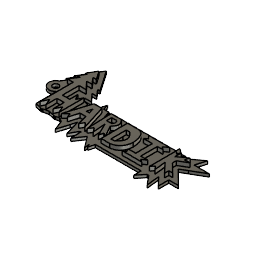
hackclub_day3 (Autodesk Fusion 360 design; units mm, degrees)
part number: 2025-12-19-10-28-26-184
Autodesk Fusion 360 part; units mm, degrees
sketch "Sketch2" plane through (0, 0, 0) normal (0, 0, 1) x (1, 0, 0)
  line L0 (23.8066, -11.3705) -> (28.9661, -18.9111)
  line L1 (28.9661, -18.9111) -> (32.7901, -24.5)
  line L2 (32.7901, -24.5) -> (30.8533, -24.5)
  line L3 (30.8533, -24.5) -> (35.4835, -29.9238)
  line L4 (35.4835, -29.9238) -> (31.3674, -29.9238)
  line L5 (31.3674, -29.9238) -> (31.9281, -30.5202)
  line L6 (31.9281, -30.5202) -> (37.5851, -36.5384)
  line L7 (37.5851, -36.5384) -> (31.3984, -36.5384)
  line L8 (31.3984, -36.5384) -> (32.4268, -38.3381)
  line L9 (32.4268, -38.3381) -> (32.6557, -38.739)
  line L10 (32.6557, -38.739) -> (38.0566, -40.1103)
  line L11 (38.0566, -40.1103) -> (38.0566, -44.6386)
  line L12 (38.0566, -44.6386) -> (39.8071, -39.0438)
  line L13 (39.8071, -39.0438) -> (40.5908, -36.5384)
  line L14 (40.5908, -36.5384) -> (45.497, -36.5384)
  line L15 (45.497, -36.5384) -> (46.8807, -31.8775)
  line L16 (46.8807, -31.8775) -> (48.1917, -36.5384)
  line L17 (48.1917, -36.5384) -> (52.7203, -36.5384)
  line L18 (52.7203, -36.5384) -> (53.504, -39.0438)
  line L19 (53.504, -39.0438) -> (54.5409, -42.3579)
  line L20 (54.5409, -42.3579) -> (54.4632, -40.2418)
  line L21 (54.4632, -40.2418) -> (54.3269, -36.5384)
  line L22 (54.3269, -36.5384) -> (68.5789, -36.5384)
  line L23 (68.5789, -36.5384) -> (68.7483, -36.7197)
  line L24 (68.7483, -36.7197) -> (68.7483, -36.5384)
  line L25 (68.7483, -36.5384) -> (79.7116, -36.5384)
  spline S0 degree 3 poles (79.7116, -36.5384) (80.9546, -36.4376) (82.1108, -36.5411) (83.1757, -36.8107) knots 0 0 0 0 1 1 1 1
  line L26 (83.1757, -36.8107) -> (82.9429, -36.5384)
  line L27 (82.9429, -36.5384) -> (110.6847, -36.5384)
  line L28 (110.6847, -36.5384) -> (110.6847, -33.1248)
  line L29 (110.6847, -33.1248) -> (115.4115, -36.5384)
  line L30 (115.4115, -36.5384) -> (119.5483, -36.5384)
  line L31 (119.5483, -36.5384) -> (117.5189, -38.0603)
  line L32 (117.5189, -38.0603) -> (117.8817, -38.3222)
  line L33 (117.8817, -38.3222) -> (120.0325, -38.83)
  line L34 (120.0325, -38.83) -> (123.5387, -36.2913)
  line L35 (123.5387, -36.2913) -> (131.9062, -30.2321)
  line L36 (131.9062, -30.2321) -> (129.3109, -39.3166)
  line L37 (129.3109, -39.3166) -> (142.5043, -39.3166)
  line L38 (142.5043, -39.3166) -> (130.9952, -45.9798)
  line L39 (130.9952, -45.9798) -> (125.3969, -49.2207)
  line L40 (125.3969, -49.2207) -> (131.7088, -55.4217)
  line L41 (131.7088, -55.4217) -> (137.9379, -61.5416)
  line L42 (137.9379, -61.5416) -> (129.4701, -61.5416)
  line L43 (129.4701, -61.5416) -> (129.4701, -70.7065)
  line L44 (129.4701, -70.7065) -> (123.2927, -64.117)
  line L45 (123.2927, -64.117) -> (122.6426, -63.4238)
  line L46 (122.6426, -63.4238) -> (123.8417, -74.6641)
  line L47 (123.8417, -74.6641) -> (117.3266, -66.7009)
  line L48 (117.3266, -66.7009) -> (115.9494, -66.7009)
  line L49 (115.9494, -66.7009) -> (110.6847, -73.1356)
  line L50 (110.6847, -73.1356) -> (110.6847, -66.7009)
  line L51 (110.6847, -66.7009) -> (71.0409, -66.7009)
  line L52 (71.0409, -66.7009) -> (69.7045, -72.0471)
  line L53 (69.7045, -72.0471) -> (68.3324, -69.2359)
  line L54 (68.3324, -69.2359) -> (68.7086, -73.7476)
  line L55 (68.7086, -73.7476) -> (61.4852, -64.1165)
  line L56 (61.4852, -64.1165) -> (55.6583, -72.7043)
  line L57 (55.6583, -72.7043) -> (55.3135, -63.3428)
  line L58 (55.3135, -63.3428) -> (54.4314, -63.8315)
  line L59 (54.4314, -63.8315) -> (50.4209, -70.8501)
  line L60 (50.4209, -70.8501) -> (48.1118, -62.6412)
  line L61 (48.1118, -62.6412) -> (46.695, -57.6032)
  line L62 (46.695, -57.6032) -> (45.185, -62.6904)
  line L63 (45.185, -62.6904) -> (42.2312, -72.64)
  line L64 (42.2312, -72.64) -> (38.9268, -64.2289)
  line L65 (38.9268, -64.2289) -> (35.6341, -62.1964)
  line L66 (35.6341, -62.1964) -> (32.7348, -62.8216)
  line L67 (32.7348, -62.8216) -> (32.5504, -63.2095)
  line L68 (32.5504, -63.2095) -> (31.7622, -63.0314)
  line L69 (31.7622, -63.0314) -> (31.2304, -63.1463)
  line L70 (31.2304, -63.1463) -> (31.1118, -62.8843)
  line L71 (31.1118, -62.8843) -> (26.1822, -61.7704)
  line L72 (26.1822, -61.7704) -> (21.5773, -62.6674)
  line L73 (21.5773, -62.6674) -> (21.2755, -63.2711)
  line L74 (21.2755, -63.2711) -> (20.0102, -62.9724)
  line L75 (20.0102, -62.9724) -> (19.7968, -63.0142)
  line L76 (19.7968, -63.0142) -> (19.7555, -62.9124)
  line L77 (19.7555, -62.9124) -> (14.5087, -61.6738)
  line L78 (14.5087, -61.6738) -> (14.5087, -36.5384)
  line L79 (14.5087, -36.5384) -> (6.5268, -36.5384)
  line L80 (6.5268, -36.5384) -> (10.0449, -31.0412)
  line L81 (10.0449, -31.0412) -> (10.7599, -29.9238)
  line L82 (10.7599, -29.9238) -> (8.676, -29.9238)
  line L83 (8.676, -29.9238) -> (11.8231, -24.5475)
  line L84 (11.8231, -24.5475) -> (11.851, -24.5)
  line L85 (11.851, -24.5) -> (10.2979, -24.5)
  line L86 (10.2979, -24.5) -> (13.4018, -19.1385)
  line L87 (13.4018, -19.1385) -> (17.7675, -11.5979)
  line L88 (17.7675, -11.5979) -> (20.6068, -6.6938)
  line L89 (20.6068, -6.6938) -> (23.8066, -11.3705)
  spline S1 degree 3 poles (80.5222, -52.3415) (80.5257, -52.3163) (80.5257, -52.3055) (80.5259, -52.3089) knots 0 0 0 0 1 1 1 1
  spline S2 degree 3 poles (80.5259, -52.3089) (80.5257, -52.3076) (80.5246, -52.3012) (80.5222, -52.2893) knots 0 0 0 0 1 1 1 1
  line L90 (80.5222, -52.2893) -> (80.5222, -52.3415)
  circle A0 centre (19.8343, -1.9154) radius 8.0516
  circle A1 centre (19.8343, -1.9154) radius 4.4627
  constraint concentric A0 A1
extrude "Extrude1" add sketch "Sketch2" along normal blind 2.5 contours L0 L1 L2 L3 L4 L5 L6 L7 L8 L9 L10 L11 L12 L13 L14 L15 L16 L17 L18 L19 L20 L21 L22 L23 L24 L25 S0 L26 L27 L28 L29 L30 L31 L32 L33 L34 L35 L36 L37 L38 L39 L40 L41 L42 L43 L44 L45 L46 L47 L48 L49 L50 L51 L52 L53 L54 L55 L56 L57 L58 L59 L60 L61 L62 L63 L64 L65 L66 L67 L68 L69 L70 L71 L72 L73 L74 L75 L76 L77 L78 L79 L80 L81 L82 L83 L84 L85 L86 L87 L88 L89 A0 | L88 L89 A0 picked at (20.9602, -8.7956)
sketch "Sketch3" plane through (0, 0, 2.5) normal (0, 0, 1) x (-1, 0, 0)
  line L0 (-80.5222, 52.3415) -> (-80.5222, 52.2893)
  spline S0 degree 3 poles (-80.5222, 52.2893) (-80.5244, 52.3) (-80.5254, 52.3062) (-80.5258, 52.3083) knots -1 -1 -1 -1 -0.105948 -0.105948 -0.105948 -0.105948
  spline S1 degree 3 poles (-80.5258, 52.3083) (-80.5256, 52.309) (-80.5252, 52.32) (-80.5222, 52.3415) knots -0.853043 -0.853043 -0.853043 -0.853043 0 0 0 0
  line L1 (-20.6068, 6.6938) -> (-17.7675, 11.5979)
  line L2 (-17.7675, 11.5979) -> (-13.4018, 19.1385)
  line L3 (-13.4018, 19.1385) -> (-10.2979, 24.5)
  line L4 (-10.2979, 24.5) -> (-11.851, 24.5)
  line L5 (-11.851, 24.5) -> (-11.8231, 24.5475)
  line L6 (-11.8231, 24.5475) -> (-8.676, 29.9238)
  line L7 (-8.676, 29.9238) -> (-10.7599, 29.9238)
  line L8 (-10.7599, 29.9238) -> (-10.0449, 31.0412)
  line L9 (-10.0449, 31.0412) -> (-6.5268, 36.5384)
  line L10 (-6.5268, 36.5384) -> (-14.5087, 36.5384)
  line L11 (-14.5087, 36.5384) -> (-14.5087, 61.6738)
  line L12 (-14.5087, 61.6738) -> (-19.7555, 62.9124)
  line L13 (-19.7555, 62.9124) -> (-19.7968, 63.0142)
  line L14 (-19.7968, 63.0142) -> (-20.0102, 62.9724)
  line L15 (-20.0102, 62.9724) -> (-21.2755, 63.2711)
  line L16 (-21.2755, 63.2711) -> (-21.5773, 62.6674)
  line L17 (-21.5773, 62.6674) -> (-26.1822, 61.7704)
  line L18 (-26.1822, 61.7704) -> (-31.1118, 62.8843)
  line L19 (-31.1118, 62.8843) -> (-31.2304, 63.1463)
  line L20 (-31.2304, 63.1463) -> (-31.7622, 63.0314)
  line L21 (-31.7622, 63.0314) -> (-32.5504, 63.2095)
  line L22 (-32.5504, 63.2095) -> (-32.7348, 62.8216)
  line L23 (-32.7348, 62.8216) -> (-35.6341, 62.1964)
  line L24 (-35.6341, 62.1964) -> (-38.9268, 64.2289)
  line L25 (-38.9268, 64.2289) -> (-42.2312, 72.64)
  line L26 (-42.2312, 72.64) -> (-45.185, 62.6904)
  line L27 (-45.185, 62.6904) -> (-46.695, 57.6032)
  line L28 (-46.695, 57.6032) -> (-48.1118, 62.6412)
  line L29 (-48.1118, 62.6412) -> (-50.4209, 70.8501)
  line L30 (-50.4209, 70.8501) -> (-54.4314, 63.8315)
  line L31 (-54.4314, 63.8315) -> (-55.3135, 63.3428)
  line L32 (-55.3135, 63.3428) -> (-55.6583, 72.7043)
  line L33 (-55.6583, 72.7043) -> (-61.4852, 64.1165)
  line L34 (-61.4852, 64.1165) -> (-68.7086, 73.7476)
  line L35 (-68.7086, 73.7476) -> (-68.3324, 69.2359)
  line L36 (-68.3324, 69.2359) -> (-69.7045, 72.0471)
  line L37 (-69.7045, 72.0471) -> (-71.0409, 66.7009)
  line L38 (-71.0409, 66.7009) -> (-110.6847, 66.7009)
  line L39 (-110.6847, 66.7009) -> (-110.6847, 73.1356)
  line L40 (-110.6847, 73.1356) -> (-115.9494, 66.7009)
  line L41 (-115.9494, 66.7009) -> (-117.3266, 66.7009)
  line L42 (-117.3266, 66.7009) -> (-123.8417, 74.6641)
  line L43 (-123.8417, 74.6641) -> (-122.6426, 63.4238)
  line L44 (-122.6426, 63.4238) -> (-123.2927, 64.117)
  line L45 (-123.2927, 64.117) -> (-129.4701, 70.7065)
  line L46 (-129.4701, 70.7065) -> (-129.4701, 61.5416)
  line L47 (-129.4701, 61.5416) -> (-137.9379, 61.5416)
  line L48 (-137.9379, 61.5416) -> (-131.7088, 55.4217)
  line L49 (-131.7088, 55.4217) -> (-125.3969, 49.2207)
  line L50 (-125.3969, 49.2207) -> (-130.9952, 45.9798)
  line L51 (-130.9952, 45.9798) -> (-142.5043, 39.3166)
  line L52 (-142.5043, 39.3166) -> (-129.3109, 39.3166)
  line L53 (-129.3109, 39.3166) -> (-131.9062, 30.2321)
  line L54 (-131.9062, 30.2321) -> (-123.5387, 36.2913)
  line L55 (-123.5387, 36.2913) -> (-120.0325, 38.83)
  line L56 (-120.0325, 38.83) -> (-117.8817, 38.3222)
  line L57 (-117.8817, 38.3222) -> (-117.5189, 38.0603)
  line L58 (-117.5189, 38.0603) -> (-119.5483, 36.5384)
  line L59 (-119.5483, 36.5384) -> (-115.4115, 36.5384)
  line L60 (-115.4115, 36.5384) -> (-110.6847, 33.1248)
  line L61 (-110.6847, 33.1248) -> (-110.6847, 36.5384)
  line L62 (-110.6847, 36.5384) -> (-82.9429, 36.5384)
  line L63 (-82.9429, 36.5384) -> (-83.1757, 36.8107)
  spline S2 degree 3 poles (-83.1757, 36.8107) (-82.1108, 36.5411) (-80.9546, 36.4376) (-79.7116, 36.5384) knots -1 -1 -1 -1 0 0 0 0
  line L64 (-79.7116, 36.5384) -> (-68.7483, 36.5384)
  line L65 (-68.7483, 36.5384) -> (-68.7483, 36.7197)
  line L66 (-68.7483, 36.7197) -> (-68.5789, 36.5384)
  line L67 (-68.5789, 36.5384) -> (-54.3269, 36.5384)
  line L68 (-54.3269, 36.5384) -> (-54.4632, 40.2418)
  line L69 (-54.4632, 40.2418) -> (-54.5409, 42.3579)
  line L70 (-54.5409, 42.3579) -> (-53.504, 39.0438)
  line L71 (-53.504, 39.0438) -> (-52.7203, 36.5384)
  line L72 (-52.7203, 36.5384) -> (-48.1917, 36.5384)
  line L73 (-48.1917, 36.5384) -> (-46.8807, 31.8775)
  line L74 (-46.8807, 31.8775) -> (-45.497, 36.5384)
  line L75 (-45.497, 36.5384) -> (-40.5908, 36.5384)
  line L76 (-40.5908, 36.5384) -> (-39.8071, 39.0438)
  line L77 (-39.8071, 39.0438) -> (-38.0566, 44.6386)
  line L78 (-38.0566, 44.6386) -> (-38.0566, 40.1103)
  line L79 (-38.0566, 40.1103) -> (-32.6557, 38.739)
  line L80 (-32.6557, 38.739) -> (-32.4268, 38.3381)
  line L81 (-32.4268, 38.3381) -> (-31.3984, 36.5384)
  line L82 (-31.3984, 36.5384) -> (-37.5851, 36.5384)
  line L83 (-37.5851, 36.5384) -> (-31.9281, 30.5202)
  line L84 (-31.9281, 30.5202) -> (-31.3674, 29.9238)
  line L85 (-31.3674, 29.9238) -> (-35.4835, 29.9238)
  line L86 (-35.4835, 29.9238) -> (-30.8533, 24.5)
  line L87 (-30.8533, 24.5) -> (-32.7901, 24.5)
  line L88 (-32.7901, 24.5) -> (-28.9661, 18.9111)
  line L89 (-28.9661, 18.9111) -> (-23.8066, 11.3705)
  line L90 (-23.8066, 11.3705) -> (-20.6068, 6.6938)
  line L91 (-72.4792, 59.2482) -> (-72.4792, 40.1982)
  line L92 (-72.4792, 40.1982) -> (-80.0198, 40.1982)
  spline S3 degree 2 poles (-80.0198, 40.1982) (-88.5098, 39.3658) (-89.4125, 52.2367) knots 0 0 0 1 1 1
  spline S4 degree 2 poles (-89.4125, 52.2367) (-88.6021, 61.8591) (-80.0198, 63.217) knots 0 0 0 1 1 1
  line L93 (-80.0198, 63.217) -> (-72.4792, 63.217)
  line L94 (-72.4792, 63.217) -> (-72.4792, 59.2482)
  line L95 (-77.1094, 45.8867) -> (-77.1094, 59.2482)
  line L96 (-77.1094, 59.2482) -> (-80.0198, 59.2482)
  spline S5 degree 2 poles (-80.0198, 59.2482) (-84.3965, 55.4321) (-84.2531, 52.2367) knots 0 0 0 1 1 1
  spline S6 degree 2 poles (-84.2531, 52.2367) (-84.1195, 49.2594) (-80.0198, 45.8867) knots 0 0 0 1 1 1
  line L97 (-80.0198, 45.8867) -> (-77.1094, 45.8867)
  line L98 (-58.9854, 61.7617) -> (-58.1917, 40.1982)
  line L99 (-58.1917, 40.1982) -> (-67.1875, 40.1982)
  spline S7 degree 3 poles (-67.1875, 40.1982) (-71.0724, 44.3532) (-70.7898, 46.4784) (-67.1875, 49.8555) knots 0 0 0 0 1 1 1 1
  line L100 (-67.1875, 49.8555) -> (-72.4792, 59.2482)
  line L101 (-72.4792, 59.2482) -> (-69.7011, 58.0576)
  line L102 (-69.7011, 58.0576) -> (-68.775, 61.7617)
  line L103 (-68.775, 61.7617) -> (-63.3511, 50.6492)
  line L104 (-63.3511, 50.6492) -> (-64.2771, 61.7617)
  line L105 (-64.2771, 61.7617) -> (-61.499, 58.0576)
  line L106 (-61.499, 58.0576) -> (-58.9854, 61.7617)
  line L107 (-61.499, 42.9763) -> (-61.499, 47.342)
  line L108 (-61.499, 47.342) -> (-65.8646, 47.342)
  spline S8 degree 3 poles (-65.8646, 47.342) (-67.5836, 45.637) (-67.3497, 44.6813) (-65.8646, 42.9763) knots 0 0 0 0 1 1 1 1
  line L109 (-65.8646, 42.9763) -> (-61.499, 42.9763)
  line L110 (-43.375, 40.1982) -> (-36.6281, 61.7617)
  line L111 (-36.6281, 61.7617) -> (-40.4646, 58.0576)
  line L112 (-40.4646, 58.0576) -> (-41.9198, 61.7617)
  line L113 (-41.9198, 61.7617) -> (-44.4333, 53.2951)
  line L114 (-44.4333, 53.2951) -> (-49.3281, 53.2951)
  line L115 (-49.3281, 53.2951) -> (-51.7094, 61.7617)
  line L116 (-51.7094, 61.7617) -> (-53.8261, 58.0576)
  line L117 (-53.8261, 58.0576) -> (-57.0011, 61.7617)
  line L118 (-57.0011, 61.7617) -> (-50.2542, 40.1982)
  line L119 (-50.2542, 40.1982) -> (-43.375, 40.1982)
  line L120 (-46.9469, 44.8284) -> (-45.6901, 49.0617)
  line L121 (-45.6901, 49.0617) -> (-48.1375, 49.0617)
  line L122 (-48.1375, 49.0617) -> (-46.9469, 44.8284)
  line L123 (-18.2396, 40.1982) -> (-18.2396, 33.0545)
  line L124 (-18.2396, 33.0545) -> (-13.2125, 33.0545)
  line L125 (-13.2125, 33.0545) -> (-17.4458, 26.4399)
  line L126 (-17.4458, 26.4399) -> (-15.0646, 26.4399)
  line L127 (-15.0646, 26.4399) -> (-18.2396, 21.0159)
  line L128 (-18.2396, 21.0159) -> (-16.6521, 21.0159)
  line L129 (-16.6521, 21.0159) -> (-21.0177, 13.4753)
  line L130 (-21.0177, 13.4753) -> (-26.1771, 21.0159)
  line L131 (-26.1771, 21.0159) -> (-23.2667, 21.0159)
  line L132 (-23.2667, 21.0159) -> (-27.8969, 26.4399)
  line L133 (-27.8969, 26.4399) -> (-23.2667, 26.4399)
  line L134 (-23.2667, 26.4399) -> (-29.4844, 33.0545)
  line L135 (-29.4844, 33.0545) -> (-23.2667, 33.0545)
  line L136 (-23.2667, 33.0545) -> (-23.2667, 40.1982)
  line L137 (-23.2667, 40.1982) -> (-23.2667, 47.342)
  line L138 (-23.2667, 47.342) -> (-29.4844, 47.342)
  line L139 (-29.4844, 47.342) -> (-29.4844, 40.1982)
  line L140 (-29.4844, 40.1982) -> (-32.1302, 44.8284)
  line L141 (-32.1302, 44.8284) -> (-34.6438, 40.1982)
  line L142 (-34.6438, 40.1982) -> (-34.6438, 61.7617)
  line L143 (-34.6438, 61.7617) -> (-32.1302, 56.2055)
  line L144 (-32.1302, 56.2055) -> (-29.4844, 61.7617)
  line L145 (-29.4844, 61.7617) -> (-29.4844, 52.2367)
  line L146 (-29.4844, 52.2367) -> (-23.2667, 52.2367)
  line L147 (-23.2667, 52.2367) -> (-23.2667, 61.7617)
  line L148 (-23.2667, 61.7617) -> (-21.0177, 56.2055)
  line L149 (-21.0177, 56.2055) -> (-18.2396, 61.7617)
  line L150 (-18.2396, 61.7617) -> (-18.2396, 40.1982)
  line L151 (-93.249, 61.7617) -> (-91.9261, 59.2482)
  line L152 (-91.9261, 59.2482) -> (-98.5406, 59.2482)
  line L153 (-98.5406, 59.2482) -> (-98.5406, 44.8284)
  line L154 (-98.5406, 44.8284) -> (-90.8677, 44.8284)
  line L155 (-90.8677, 44.8284) -> (-93.249, 42.9763)
  line L156 (-93.249, 42.9763) -> (-90.8677, 40.1982)
  line L157 (-90.8677, 40.1982) -> (-108.9917, 40.1982)
  line L158 (-108.9917, 40.1982) -> (-105.2875, 42.9763)
  line L159 (-105.2875, 42.9763) -> (-107.8011, 44.8284)
  line L160 (-107.8011, 44.8284) -> (-102.9063, 44.8284)
  line L161 (-102.9063, 44.8284) -> (-102.9063, 59.2482)
  line L162 (-102.9063, 59.2482) -> (-108.9917, 59.2482)
  line L163 (-108.9917, 59.2482) -> (-105.2875, 61.7617)
  line L164 (-105.2875, 61.7617) -> (-107.8011, 63.217)
  line L165 (-107.8011, 63.217) -> (-90.8677, 63.217)
  line L166 (-90.8677, 63.217) -> (-93.249, 61.7617)
  line L167 (-114.4156, 63.217) -> (-114.4156, 40.1982)
  line L168 (-114.4156, 40.1982) -> (-116.7969, 41.918)
  line L169 (-116.7969, 41.918) -> (-118.1198, 39.2722)
  line L170 (-118.1198, 39.2722) -> (-118.1198, 44.8284)
  line L171 (-118.1198, 44.8284) -> (-125.7927, 39.2722)
  line L172 (-125.7927, 39.2722) -> (-124.7344, 42.9763)
  line L173 (-124.7344, 42.9763) -> (-129.3646, 42.9763)
  line L174 (-129.3646, 42.9763) -> (-121.824, 47.342)
  line L175 (-121.824, 47.342) -> (-121.824, 50.6492)
  line L176 (-121.824, 50.6492) -> (-129.3646, 58.0576)
  line L177 (-129.3646, 58.0576) -> (-126.0573, 58.0576)
  line L178 (-126.0573, 58.0576) -> (-126.0573, 61.7617)
  line L179 (-126.0573, 61.7617) -> (-118.1198, 53.2951)
  line L180 (-118.1198, 53.2951) -> (-119.1781, 63.217)
  line L181 (-119.1781, 63.217) -> (-116.7969, 60.3065)
  line L182 (-116.7969, 60.3065) -> (-114.4156, 63.217)
extrude "Extrude2" add sketch "Sketch3" along normal blind 3.5 contours L0 S0 S1 | L91 L92 S3 S4 L93 L94 | L98 L99 S7 L100 L101 L102 L103 L104 L105 L106 | L110 L111 L112 L113 L114 L115 L116 L117 L118 L119 | L123 L124 L125 L126 L127 L128 L129 L130 L131 L132 L133 L134 L135 L136 L137 L138 L139 L140 L141 L142 L143 L144 L145 L146 L147 L148 L149 L150 | L151 L152 L153 L154 L155 L156 L157 L158 L159 L160 L161 L162 L163 L164 L165 L166 | L167 L168 L169 L170 L171 L172 L173 L174 L175 L176 L177 L178 L179 L180 L181 L182
sketch "Sketch5" plane through (0, 0, 0) normal (0, 0, 1) x (1, 0, 0)
  circle A0 centre (10, -40) radius 5.8684
  circle A1 centre (10, -40) radius 2.5225
  constraint concentric A0 A1
extrude "Extrude3" add sketch "Sketch5" along normal blind 2.2
extrude "Extrude4" add 1 faces at (13.8467, -40.0982, 2.2) along direction (0, 0, 1) blind 0.3
